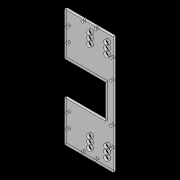
# Autodesk Inventor part: AdaptivePrintedLid
Saved by Autodesk Inventor 2022 (Build 260153000, 153)
## iProperties
Created: 2021-03-30
Part Number: AdaptivePrintedLid
Material: PBT Plastic
Document SubType Name: Modeling
Designer: Esketitttttt
Density: 1.31 g/cm^3
Appearance: Clear
Author: Esketitttttt
Autodesk Inventor part; units mm, degrees
ref_plane "YZ Plane" through (0, 0, 0) normal (1, 0, 0) x (0, 1, 0)
ref_plane "XZ Plane" through (0, 0, 0) normal (0, 1, 0) x (-1, 0, 0)
ref_plane "Work Plane1" through (0, -4.7625, 0) normal (0, 0, 1) x (1, 0, 0)
sketch "Sketch1" plane through (0, -4.7625, 0) normal (0, 0, 1) x (1, 0, 0)
  circle A0 centre (-57.1962, 44.0311) radius 1.4732
  circle A1 centre (-57.1962, 63.0811) radius 1.4732
  circle A2 centre (0.7938, -21.5437) radius 1.4732 projected
  circle A3 centre (0.7938, 56.2124) radius 1.4732
  circle A4 centre (-57.1962, -54.6144) radius 1.4732
  circle A5 centre (0.7938, 30.2937) radius 1.4732
  circle A6 centre (-57.1962, -35.5644) radius 1.4732 projected
  circle A7 centre (-36.8079, -70.2061) radius 0.762
  circle A8 centre (-19.5946, -70.2061) radius 0.762
  line L0 (3.9688, -73.3811) -> (3.9688, 82.1311) projected
  line L1 (3.9688, 82.1311) -> (-54.0212, 82.1311) projected
  line L2 (-54.0212, 24.9811) -> (-60.3712, 24.9811) projected
  line L3 (-2.3812, 75.7811) -> (-54.0212, 75.7811) projected
  line L4 (-2.3812, 75.7811) -> (-2.3812, -67.0311) projected
  line L5 (-54.0212, -67.0311) -> (-2.3812, -67.0311) projected
  line L6 (-60.3712, -16.2311) -> (-54.0212, -16.2311) projected
  line L7 (3.9688, -73.3811) -> (-54.0212, -73.3811) projected
  line L8 (-6.0508, 24.9811) -> (-6.0508, 18.6311) projected
  line L9 (-6.0507, -9.8811) -> (-6.0507, -16.2311) projected
  line L10 (-6.0507, -16.2311) -> (-54.0212, -16.2311)
  line L11 (-54.0212, 24.9811) -> (-6.0508, 24.9811)
  line L12 (-6.0508, 24.9811) -> (-6.0507, -16.2311)
  circle A9 centre (0.7938, -21.5437) radius 1.7907
  circle A10 centre (-19.5946, -70.2061) radius 1.7907
  circle A11 centre (-36.8079, -70.2061) radius 1.7907
  circle A12 centre (-57.1962, -54.6144) radius 1.7907
  circle A13 centre (-57.1962, -35.5644) radius 1.7907
  circle A14 centre (-57.1962, 44.0311) radius 1.7907
  circle A15 centre (-57.1962, 63.0811) radius 1.7907
  circle A16 centre (-36.8079, 78.9561) radius 1.7907
  circle A17 centre (-19.5946, 78.9561) radius 1.7907
  circle A18 centre (0.7938, 56.2124) radius 1.7907
  circle A19 centre (0.7938, 30.2937) radius 1.7907
  circle A20 centre (18.1645, 33.6336) radius 1.75
  circle A21 centre (40.5905, 33.6336) radius 1.75
  circle A22 centre (40.5905, 40.5086) radius 1.75
  circle A23 centre (40.5905, 26.7586) radius 1.75
  circle A24 centre (18.1645, 40.5086) radius 1.75
  circle A25 centre (18.1645, 26.7586) radius 1.75
  line L13 (43.7675, 21.6336) -> (43.7675, 45.6336)
  line L14 (14.9875, 45.6336) -> (43.7675, 45.6336)
  line L15 (14.9875, 21.6336) -> (14.9875, 45.6336)
  line L16 (43.7675, 21.6336) -> (14.9875, 21.6336)
  circle A26 centre (-27.9842, 63.7811) radius 1.75
  circle A27 centre (-5.5583, 63.7811) radius 1.75
  circle A28 centre (-5.5583, 70.6561) radius 1.75
  circle A29 centre (-5.5583, 56.9061) radius 1.75
  circle A30 centre (-27.9842, 70.6561) radius 1.75
  circle A31 centre (-27.9842, 56.9061) radius 1.75
  line L17 (-2.3812, 51.7811) -> (-2.3812, 75.7811)
  line L18 (-31.1612, 75.7811) -> (-2.3812, 75.7811)
  line L19 (-31.1612, 51.7811) -> (-31.1612, 75.7811)
  line L20 (-2.3812, 51.7811) -> (-31.1612, 51.7811)
  circle A32 centre (-5.5583, 70.6561) radius 3.175
  circle A33 centre (-5.5583, 63.7811) radius 3.175
  circle A34 centre (-5.5583, 56.9061) radius 3.175
  circle A35 centre (-27.9842, 56.9061) radius 3.175
  circle A36 centre (-27.9842, 63.7811) radius 3.175
  circle A37 centre (-27.9842, 70.6561) radius 3.175
  line L21 (-54.0212, 94.8311) -> (-54.0212, 82.1311) projected
  line L22 (-60.3712, 94.8311) -> (-54.0212, 94.8311) projected
  line L23 (-60.3712, 24.9811) -> (-60.3712, 94.8311) projected
  line L24 (-54.0212, 75.7811) -> (-54.0212, 24.9811) projected
  line L25 (-54.0212, -16.2311) -> (-54.0212, -67.0311) projected
  line L26 (-60.3712, -86.0811) -> (-60.3712, -16.2311) projected
  line L27 (-54.0212, -86.0811) -> (-60.3712, -86.0811) projected
  line L28 (-54.0212, -73.3811) -> (-54.0212, -86.0811) projected
  line L29 (-54.0212, 82.1311) -> (-60.3712, 82.1311)
  line L30 (-54.0212, -73.3811) -> (-60.3712, -73.3811)
  circle A38 centre (0.7938, 56.2124) radius 1.4732 projected
  circle A39 centre (0.7938, 30.2937) radius 1.4732 projected
  circle A40 centre (-57.1962, 63.0811) radius 1.4732 projected
  circle A41 centre (-57.1962, 44.0311) radius 1.4732 projected
  circle A42 centre (-36.8079, 78.9561) radius 1.4732 projected
  circle A43 centre (-19.5946, 78.9561) radius 1.4732 projected
  circle A44 centre (-27.9842, -48.1461) radius 1.75 construction
  circle A45 centre (-27.9842, -55.0211) radius 1.75 construction
  circle A46 centre (-27.9842, -61.8961) radius 1.75 construction
  circle A47 centre (-5.5583, -61.8961) radius 1.75 construction
  circle A48 centre (-5.5583, -55.0211) radius 1.75 construction
  circle A49 centre (-5.5583, -48.1461) radius 1.75 construction
  circle A50 centre (-27.9842, -48.1461) radius 3.175
  circle A51 centre (-27.9842, -55.0211) radius 3.175
  circle A52 centre (-27.9842, -61.8961) radius 3.175
  circle A53 centre (-5.5583, -48.1461) radius 3.175
  circle A54 centre (-5.5583, -55.0211) radius 3.175
  circle A55 centre (-5.5583, -61.8961) radius 3.175
  circle A56 centre (0.7938, -47.4624) radius 1.4732 projected
  circle A57 centre (0.7938, -47.4624) radius 1.4732 projected
  circle A58 centre (0.7938, -47.4624) radius 1.7907
  line L31 (-2.3812, -67.0311) -> (-2.3812, -73.3811) construction
  line L32 (-60.3712, -16.2311) -> (-6.0507, -16.2311)
  line L33 (-6.0507, -16.2311) -> (-6.0507, -19.4061)
  line L34 (-6.0507, -19.4061) -> (-60.3712, -19.4061)
  line L35 (-60.3712, -19.4061) -> (-60.3712, -16.2311)
  point P0 (29.6789, 33.6336)
  point P1 (-16.4699, 63.7811)
  point P2 (-2.3812, -70.2061)
  dimension "o" = 0.3175
  dimension "d38" = 0.3175
  dimension "d39" = 0.3175
  dimension "d40" = 0.3175
  dimension "d41" = 0.3175
  dimension "d44" = 0.3175
  dimension "d45" = 0.3175
  dimension "d46" = 6.35
  dimension "d47" = 6.35
  dimension "d48" = 6.35
  dimension "d49" = 6.35
  dimension "d50" = 6.35
  dimension "d51" = 6.35
  dimension "d58" = 3.5814
  dimension "d59" = 3.5814
  dimension "d60" = 3.5814
  dimension "d61" = 3.5814
  dimension "d62" = 3.5814
  dimension "d63" = 6.35
  dimension "d64" = 6.35
  dimension "d65" = 6.35
  dimension "d66" = 6.35
  dimension "d67" = 6.35
  dimension "d68" = 6.35
  dimension "d69" = 0.3175
  dimension "d70" = 19.05
  dimension "d71" = 19.05
  dimension "d72" = 2.9464
  dimension "d73" = 3.5814
  dimension "d74" = 2.9464
  dimension "d75" = 3.175
  constraints: 43 centre point, 36 end point, 18 coincident, 4 concentric, 4 vertical alignment, 3 horizontal, 3 parallel, 3 perpendicular, 2 horizontal alignment, 2 point on line, 1 midpoint, 6 other
  measures "o" radial gap between concentric circles of A2 A9
  measures "d38" radial gap between concentric circles of A4 A12
  measures "d39" radial gap between concentric circles of A6 A13
  measures "d40" radial gap between concentric circles of A0 A14
  measures "d41" radial gap between concentric circles of A1 A15
  measures "d44" radial gap between concentric circles of A3 A18
  measures "d45" radial gap between concentric circles of A5 A19
  measures "d46" diameter of A32
  measures "d47" diameter of A33
  measures "d48" diameter of A34
  measures "d49" diameter of A35
  measures "d50" diameter of A36
  measures "d51" diameter of A37
  measures "d58" diameter of A9
  measures "d59" diameter of A17
  measures "d60" diameter of A16
  measures "d61" diameter of A11
  measures "d62" diameter of A10
  measures "d63" diameter of A50
  measures "d64" diameter of A51
  measures "d65" diameter of A52
  measures "d66" diameter of A53
  measures "d67" diameter of A54
  measures "d68" diameter of A55
  measures "d69" radial gap between concentric circles of A56 A58
  measures "d70" distance of A0.centre A1.centre
  measures "d71" distance of A6.centre A4.centre
  measures "d72" diameter of A6
  measures "d73" diameter of A13
  measures "d74" diameter of A4
  measures "d75" distance between parallel lines of L34 L10
extrude "Extrusion1" add sketch "Sketch1" along normal blind 3.175 from surface at 0 contours L7 L30 L26 L34 L25 L5 L4 L3 L24 L2 L23 L29 L1 L0 | L34 L33 L9 L12 L8 L11 L24 L3 L19 L20 L4 L5 L25 | L3 L4 L20 L19
equation "\"d38\" = o"
equation "\"d39\" = o"
equation "\"d40\" = o"
equation "\"d41\" = o"
equation "\"d44\" = o"
equation "\"d45\" = o"
body "Solid1"
